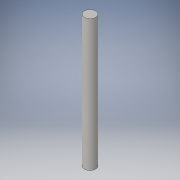
# Autodesk Inventor part: Welle
Saved by Autodesk Inventor 2016 (Build 200138000, 138)
## iProperties
Created: 2017-10-13
Part Number: Welle
Material: Generisch
Document SubType Name: Modeling
Designer: Dominik
Density: 1 g/cm^3
Appearance: Vorgabe
Author: Dominik
Autodesk Inventor part; units mm, degrees
ref_plane "YZ Plane" through (0, 0, 0) normal (1, 0, 0) x (0, 1, 0)
ref_plane "XZ Plane" through (0, 0, 0) normal (0, 1, 0) x (-1, 0, 0)
ref_plane "XY Plane" through (0, 0, 0) normal (0, 0, 1) x (1, 0, 0)
sketch "Skizze1" plane through (0, 0, 0) normal (0, 0, 1) x (1, 0, 0)
  circle A0 centre (0, 0) radius 15
  dimension "d0" = 30
  constraints: 1 centre point, 1 coincident
  measures "d0" diameter of A0
extrude "Extrusion1" add sketch "Skizze1" along normal blind 350
